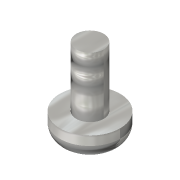
# Autodesk Inventor part: screw
Saved by Autodesk Inventor 2016 SP1 (Build 200210100, 210)
## iProperties
Created: 2018-07-05
Part Number: screw
Material: Stahl
Document SubType Name: Modeling
Designer: WhoTheHeck
Density: 7.85 g/cm^3
Appearance: Poliert - gebürstet
Author: WhoTheHeck
Autodesk Inventor part; units mm, degrees
ref_plane "YZ Plane" through (0, 0, 0) normal (1, 0, 0) x (0, 1, 0)
ref_plane "XZ Plane" through (0, 0, 0) normal (0, 1, 0) x (-1, 0, 0)
ref_plane "XY Plane" through (0, 0, 0) normal (0, 0, 1) x (1, 0, 0)
sketch "Skizze1" plane through (0, 0, 0) normal (0, 0, 1) x (1, 0, 0)
  circle A0 centre (0, 0) radius 1.65
  dimension "d0" = 3.3
  constraints: 1 centre point, 1 coincident
  measures "d0" diameter of A0
extrude "Extrusion1" add sketch "Skizze1" along normal blind 1.3
sketch "Skizze2" plane through (0, 0, 1.3) normal (0, 0, 1) x (1, 0, 0)
  circle A0 centre (0, 0) radius 0.75
  dimension "d3" = 1.5
  constraints: 1 centre point, 1 coincident
  measures "d3" diameter of A0
extrude "Extrusion2" add sketch "Skizze2" along normal blind 3.3
sketch "Skizze3" plane through (0, 0, 0) normal (0, 0, -1) x (-1, 0, 0)
  line L0 (-0.275, -1.2) -> (0.275, -1.2)
  line L1 (0.275, -1.2) -> (0.275, 1.2)
  line L2 (0.275, 1.2) -> (-0.275, 1.2)
  line L3 (-0.275, 1.2) -> (-0.275, -1.2)
  line L4 (-0.275, -1.2) -> (0.275, 1.2) construction
  line L5 (0.275, -1.2) -> (-0.275, 1.2) construction
  line L6 (-1.2, -0.275) -> (1.2, -0.275)
  line L7 (1.2, -0.275) -> (1.2, 0.275)
  line L8 (1.2, 0.275) -> (-1.2, 0.275)
  line L9 (-1.2, 0.275) -> (-1.2, -0.275)
  line L10 (-1.2, -0.275) -> (1.2, 0.275) construction
  line L11 (1.2, -0.275) -> (-1.2, 0.275) construction
  point P0 (0, 0)
  dimension "d6" = 0.55
  dimension "d7" = 0.55
  dimension "d8" = 2.4
  dimension "d9" = 2.4
  constraints: 24 end point, 4 midpoint, 4 parallel, 2 horizontal, 2 perpendicular
  measures "d6" distance of L1.end L2.end
  measures "d7" distance of L6.end L7.end
  measures "d8" distance of L7.end L8.end
  measures "d9" distance of L0.end L1.end
extrude "Extrusion3" cut sketch "Skizze3" against normal blind 1
fillet "Rundung1" radius 0.8 1 edges at (-1.65, 0, 0)
equation "\"d7\" = d6"
